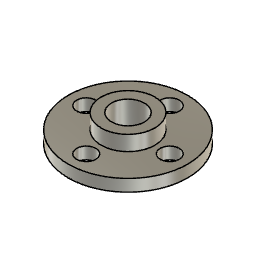
金属舵盘 v4 (Autodesk Fusion 360 design; units mm, degrees)
Autodesk Fusion 360 part; units mm, degrees
sketch "草图1" plane through (0, 0, 0) normal (0, 0, 1) x (1, 0, 0)
  circle A0 centre (0, 0) radius 10
  circle A1 centre (0, 0) radius 7 construction
  line L0 (-4, 0) -> (3, 0)
  circle A2 centre (7, 0) radius 1.6
  circle A3 centre (0, 7) radius 1.6
  circle A4 centre (-7, 0) radius 1.6
  circle A5 centre (0, -7) radius 1.6
  dimension "d1" = 20
  dimension "d2" = 14
  dimension "d3" = 3.2
  dimension "d5" = 360
  constraint coincident A0.centre A1.centre
  constraint concentric A0 A1
  constraint horizontal L0
  constraint coincident A1 A2.centre
  constraint coincident L0 A2.centre
  constraint coincident A0.centre L0
  measures "d1" diameter of A0
  measures "d2" diameter of A1
  measures "d3" diameter of A2
extrude "拉伸1" add sketch "草图1" along normal blind 2 makes body 1
sketch "草图2" plane through (0, 0, 2) normal (0, 0, 1) x (-1, 0, 0)
  circle A0 centre (0, 7) radius 1.6
  circle A1 centre (7, 0) radius 1.6
  circle A2 centre (-7, 0) radius 1.6
  circle A3 centre (0, -7) radius 1.6
  circle A4 centre (0, 0) radius 10
  circle A5 centre (0, 0) radius 4.5
  dimension "d8" = 9
  constraint concentric A4 A5
  measures "d8" diameter of A5
extrude "拉伸2" add sketch "草图2" along normal blind 2.5 contours A5 bodies 1
sketch "草图3" plane through (0, 0, 4.5) normal (0, 0, 1) x (-1, 0, 0)
  circle A0 centre (0, 0) radius 4.5
  circle A1 centre (0, 0) radius 2.75
  dimension "d11" = 5.5
  constraint coincident A0.centre A1.centre
  measures "d11" diameter of A1
extrude "拉伸3" cut sketch "草图3" against normal blind 4 contours A1 bodies 1
sketch "草图4" plane through (0, 0, 0.5) normal (0, 0, 1) x (-1, 0, 0)
  circle A0 centre (0, 0) radius 2.75
  circle A1 centre (0, 0) radius 1.6
  dimension "d14" = 3.2
  constraint coincident A0.centre A1.centre
  measures "d14" diameter of A1
extrude "拉伸4" cut sketch "草图4" against normal blind 2 contours A1 bodies 1
copy_body "实体->零部件1" bodies 1 removing the originals makes body 2 in component "金属舵盘"
component "金属舵盘" placed x (1, 0, 0) y (0, 1, 0) z (0, 0, 1) at (0, 0, 0)
